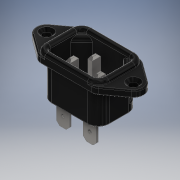
# Autodesk Inventor part: IEC C14
Saved by Autodesk Inventor 2017 SP1 (Build 210196100, 196)
## iProperties
Created: 2012-02-15
Part Number: IEC C14
Material: Tworzywo sztuczne, nieprzezroczyste czarne
Document SubType Name: Modeling
Designer: Ioannis
Density: 0.952 g/cm^3
Appearance: Gładkie - czarne
Author: Ioannis
Autodesk Inventor part; units mm, degrees
ref_plane "YZ Plane" through (0, 0, 0) normal (1, 0, 0) x (0, 1, 0)
ref_plane "XZ Plane" through (0, 0, 0) normal (0, 1, 0) x (-1, 0, 0)
ref_plane "XY Plane" through (0, 0, 0) normal (0, 0, 1) x (1, 0, 0)
sketch "Block1" plane through (0, 0, 0) normal (0, 0, 1) x (1, 0, 0)
  line L0 (24.7204, 7.7183) -> (30.7204, 7.7183)
  line L1 (30.7204, 7.7183) -> (30.7204, 9.1183)
  line L2 (29.2204, 14.6183) -> (26.2204, 14.6183)
  line L3 (24.7204, 9.1183) -> (24.7204, 7.7183)
  line L4 (26.2204, 14.6183) -> (24.7204, 9.1183)
  line L5 (30.7204, 9.1183) -> (29.2204, 14.6183)
  point P0 (27.9704, 11.8933)
  point P1 (30.7204, 14.6183)
  point P2 (24.7204, 14.6183)
  dimension "d122" = 6
  dimension "d123" = 6.9
  dimension "d124" = 1.5
  dimension "d125" = 5.5
  dimension "d126" = 5.5
  dimension "d127" = 1.5
  dimension "d128" = 6
  dimension "d130" = 105.255
  dimension "d131" = 105.255
  dimension "d132" = 1.4
  dimension "d133" = 1.4
  measures "d122" distance of point (24.72, 14.618) point (30.72, 14.618)
  measures "d123" distance of point (30.72, 14.618) L0.end
  measures "d124" distance of L2.end point (24.72, 14.618)
  measures "d125" distance of L3.start point (24.72, 14.618)
  measures "d126" distance of L1.end point (30.72, 14.618)
  measures "d127" distance of L2.start point (30.72, 14.618)
  measures "d128" distance of L0.start L0.end
  measures "d130" angle of L4 L2
  measures "d131" angle of L5 L2
  measures "d132" distance of L3.start L0.start
  measures "d133" distance of L0.end L1.end
sketch "Sketch1" plane through (0, 0, 0) normal (0, 0, 1) x (1, 0, 0)
  line L0 (-24.75, -11) -> (24.75, -11) construction
  line L1 (24.75, -11) -> (24.75, 11) construction
  line L2 (24.75, 11) -> (-24.75, 11) construction
  line L3 (-24.75, 11) -> (-24.75, -11) construction
  line L4 (-24.75, 0) -> (24.75, 0) construction
  circle A0 centre (-20, 0) radius 1.75 construction
  circle A1 centre (20, 0) radius 1.75 construction
  circle A2 centre (-20, 0) radius 4.75 construction
  circle A3 centre (20, 0) radius 4.75 construction
  line L5 (-14.0544, 10.2293) -> (-22.803, 3.8348)
  line L6 (22.803, 3.8348) -> (14.0544, 10.2293)
  line L7 (11.694, 11) -> (-11.694, 11)
  line L8 (-22.803, -3.8348) -> (-14.0544, -10.2293)
  line L9 (-11.694, -11) -> (11.694, -11)
  line L10 (14.0544, -10.2293) -> (22.803, -3.8348)
  arc A4 (-22.803, 3.8348) -> (-22.803, -3.8348) centre (-20, 0) ccw
  arc A5 (22.803, -3.8348) -> (22.803, 3.8348) centre (20, 0) ccw
  arc A6 (-11.694, 11) -> (-14.0544, 10.2293) centre (-11.694, 7) ccw
  arc A7 (14.0544, 10.2293) -> (11.694, 11) centre (11.694, 7) ccw
  arc A8 (11.694, -11) -> (14.0544, -10.2293) centre (11.694, -7) ccw
  arc A9 (-14.0544, -10.2293) -> (-11.694, -11) centre (-11.694, -7) ccw
  line L11 (9.875, -11) -> (-9.875, -11)
  line L12 (-14.875, -6) -> (-14.875, 6)
  line L13 (-9.875, 11) -> (9.875, 11)
  line L14 (14.875, 6) -> (14.875, -6)
  line L15 (9.875, -8.2) -> (-9.875, -8.2)
  line L16 (-12.075, -6) -> (-12.075, 6)
  line L17 (-9.875, 8.2) -> (9.875, 8.2)
  line L18 (12.075, 6) -> (12.075, -6)
  arc A10 (-9.875, 11) -> (-14.875, 6) centre (-9.875, 6) ccw
  arc A11 (14.875, 6) -> (9.875, 11) centre (9.875, 6) ccw
  arc A12 (-14.875, -6) -> (-9.875, -11) centre (-9.875, -6) ccw
  arc A13 (9.875, -11) -> (14.875, -6) centre (9.875, -6) ccw
  arc A14 (-9.875, 8.2) -> (-12.075, 6) centre (-9.875, 6) ccw
  arc A15 (12.075, 6) -> (9.875, 8.2) centre (9.875, 6) ccw
  arc A16 (9.875, -8.2) -> (12.075, -6) centre (9.875, -6) ccw
  arc A17 (-12.075, -6) -> (-9.875, -8.2) centre (-9.875, -6) ccw
  line L19 (-12.075, 6) -> (-9.875, 8.2)
  line L20 (12.075, 6) -> (9.875, 8.2)
  point P0 (0, 0)
  point P1 (0, 11)
  point P2 (13, 11)
  point P3 (-13, 11)
  point P4 (0, 11)
  point P5 (-13, -11)
  point P6 (13, -11)
  point P7 (0, -11)
  point P8 (0, -11)
  point P9 (0, 11)
  point P10 (14.875, 0)
  dimension "d0" = 49.5
  dimension "d1" = 22
  dimension "d2" = 3.5
  dimension "d3" = 3.5
  dimension "d4" = 4.75
  dimension "d5" = 4.75
  dimension "d6" = 40
  dimension "d7" = 26
  dimension "d8" = 26
  dimension "d9" = 4
  dimension "d10" = 4
  dimension "d11" = 4
  dimension "d12" = 4
  dimension "d13" = 2.8
  dimension "d14" = 5
  dimension "d15" = 5
  dimension "d16" = 2.2
  dimension "d17" = 2.2
  dimension "d18" = 2.2
  dimension "d19" = 2.2
  dimension "d20" = 29.75
  dimension "d21" = 24.15
  constraints: 42 end point, 34 point on circle, 28 tangent, 18 centre point, 10 perpendicular, 10 point on line, 8 midpoint, 6 coincident, 3 collinear, 2 equal radius, 2 horizontal, 2 horizontal alignment, 2 parallel, 2 vertical alignment, 3 other
  measures "d0" distance of L1.end L2.end
  measures "d1" distance of L2.end L0.start
  measures "d2" diameter of A1
  measures "d3" diameter of A0
  measures "d4" distance from line of L3 A0.centre
  measures "d5" distance from line of L1 A1.centre
  measures "d6" distance of A1.centre A0.centre
  measures "d7" distance of point (13, 11) point (-13, 11)
  measures "d8" distance of point (-13, -11) point (13, -11)
  measures "d9" radius of A6
  measures "d10" radius of A7
  measures "d11" radius of A8
  measures "d12" radius of A9
  measures "d13" distance between parallel lines of L14 L18
  measures "d14" radius of A10
  measures "d15" radius of A12
  measures "d16" radius of A14
  measures "d17" radius of A15
  measures "d18" radius of A16
  measures "d19" radius of A17
  measures "d20" distance between parallel lines of L14 L12
  measures "d21" distance between parallel lines of L18 L16
extrude "Extrusion1" add sketch "Sketch1" against normal blind 3.2 contours A6 L7 A10 L12 A12 L9 A9 L8 A4 L5 | L7 A11 L14 A13 L9 A12 L12 A10 | L7 A7 L6 A5 L10 A8 L9 A13 L14 A11 | L15 A17 L16 L19 L17 L20 L18 A16 | L20 A15 | A14 L19
extrude "Extrusion2" add sketch "Sketch1" along normal blind 1.8 contours L7 A11 L14 A13 L9 A12 L12 A10
sketch "Sketch2" plane through (0, 0, -3.2) normal (0, 0, -1) x (-1, 0, 0)
  line L0 (-12.075, -6) -> (-12.075, 6) projected
  arc A0 (-9.875, 8.2) -> (-12.075, 6) centre (-9.875, 6) ccw projected
  line L1 (-9.875, 8.2) -> (9.875, 8.2) projected
  arc A1 (12.075, 6) -> (9.875, 8.2) centre (9.875, 6) ccw projected
  line L2 (12.075, 6) -> (12.075, -6) projected
  arc A2 (9.875, -8.2) -> (12.075, -6) centre (9.875, -6) ccw projected
  line L3 (9.875, -8.2) -> (-9.875, -8.2) projected
  arc A3 (-12.075, -6) -> (-9.875, -8.2) centre (-9.875, -6) ccw projected
  line L4 (8.325, 9.45) -> (-8.325, 9.45)
  line L5 (-13.325, 4.45) -> (-13.325, -4.45)
  line L6 (-8.325, -9.45) -> (8.325, -9.45)
  line L7 (13.325, -4.45) -> (13.325, 4.45)
  arc A4 (-8.325, 9.45) -> (-13.325, 4.45) centre (-8.325, 4.45) ccw
  arc A5 (13.325, 4.45) -> (8.325, 9.45) centre (8.325, 4.45) ccw
  arc A6 (8.325, -9.45) -> (13.325, -4.45) centre (8.325, -4.45) ccw
  arc A7 (-13.325, -4.45) -> (-8.325, -9.45) centre (-8.325, -4.45) ccw
  point P0 (0, 0)
  dimension "d28" = 1.25
  dimension "d29" = 1.25
  dimension "d30" = 1.25
  dimension "d31" = 1.25
  dimension "d32" = 5
  dimension "d33" = 5
  dimension "d34" = 5
  dimension "d35" = 5
  constraints: 8 end point, 8 point on circle, 8 tangent, 4 centre point, 4 parallel
  measures "d28" distance between parallel lines of L0 L5
  measures "d29" distance between parallel lines of L4 L1
  measures "d30" distance between parallel lines of L3 L6
  measures "d31" distance between parallel lines of L2 L7
  measures "d32" radius of A4
  measures "d33" radius of A5
  measures "d34" radius of A6
  measures "d35" radius of A7
extrude "Extrusion4" add sketch "Sketch2" along normal blind 15 contours L0 A0 L1 A1 L2 A2 L3 A3 | A5 L7 A6 L6 A7 L5 A4 L4
extrude "Extrusion3" cut sketch "Sketch1" against normal blind 17.2 contours L15 A17 L16 L19 L17 L20 L18 A16 | L20 A15 | A14 L19
hole "Hole1" at (-20, 0, 0) at (20, 0, 0) direction (0, 0, -1) diameter 3.5 end through all countersink diameter 6 countersink angle 90
extrude "Extrusion5" add sketch "Sketch1" against normal up to surface (17.2 mm away) contours L20 A15 | A14 L19
move faces "Move Face1" translate (1.4142, -1.4142, 0) faces at (-11.3417, 6.7333, -5.7333) (10.6083, 7.4667, -5.7333)
move faces "Move Face2" translate (-1.4142, -1.4142, 0) faces at (10.6083, 7.4667, -5.7333)
ref_plane "Work Plane1" through (0, 0, -6.3) normal (0, 0, 1) x (1, 0, 0)
sketch "Sketch3" plane through (0, 0, -6.3) normal (0, 0, 1) x (1, 0, 0)
  line L0 (13.325, 5.125) -> (13.325, 9.45)
  line L1 (13.325, 9.45) -> (9, 9.45)
  line L2 (9, 9.45) -> (13.325, 5.125)
  line L3 (-9, 9.45) -> (-13.325, 9.45)
  line L4 (-13.325, 9.45) -> (-13.325, 5.125)
  line L5 (-13.325, 5.125) -> (-9, 9.45)
  line L6 (9, 9.45) -> (-9, 9.45) construction
  line L7 (8.325, 9.45) -> (-8.325, 9.45) construction
  line L8 (13.325, -4.45) -> (13.325, 4.45) construction
  line L9 (-13.325, 4.45) -> (-13.325, -4.45) construction
  point P0 (0, 0)
  point P1 (0, 9.45)
  dimension "d52" = 18
  dimension "d53" = 45
  dimension "d54" = 45
  constraints: 14 end point, 4 collinear, 3 perpendicular, 1 horizontal, 1 midpoint, 1 vertical, 1 vertical alignment
  measures "d52" distance of L3.start L1.end
  measures "d53" angle of L4 L5
  measures "d54" angle of L0 L2
extrude "Extrusion6" cut sketch "Sketch3" against normal blind 8
sketch "Sketch5" plane through (0, 0, -18.2) normal (0, 0, -1) x (-1, 0, 0)
  circle A0 centre (0, -2.45) radius 1.5
  arc A1 (13.325, 4.45) -> (8.325, 9.45) centre (8.325, 4.45) ccw projected
  line L0 (-8.325, 9.45) -> (8.325, 9.45) projected
  arc A2 (-8.325, 9.45) -> (-13.325, 4.45) centre (-8.325, 4.45) ccw projected
  line L1 (-13.325, -4.45) -> (-13.325, 4.45) projected
  arc A3 (-13.325, -4.45) -> (-8.325, -9.45) centre (-8.325, -4.45) ccw projected
  line L2 (8.325, -9.45) -> (-8.325, -9.45) projected
  arc A4 (8.325, -9.45) -> (13.325, -4.45) centre (8.325, -4.45) ccw projected
  line L3 (13.325, 4.45) -> (13.325, -4.45) projected
  line L4 (0, 9.45) -> (0, -9.45)
  line L5 (-7.75, 1.0821) -> (-4.75, 1.0821)
  line L6 (-4.75, 1.0821) -> (-3.75, -2.65)
  line L7 (-3.75, -2.65) -> (3.75, -2.65)
  line L8 (3.75, -2.65) -> (4.75, 1.0821)
  line L9 (4.75, 1.0821) -> (7.75, 1.0821)
  line L10 (8.325, -9.45) -> (-8.325, -9.45) projected
  line L11 (7.75, 2.5821) -> (3.599, 2.5821)
  line L12 (3.599, 2.5821) -> (2.599, -1.15)
  line L13 (2.599, -1.15) -> (-2.599, -1.15)
  line L14 (-2.599, -1.15) -> (-3.599, 2.5821)
  line L15 (-3.599, 2.5821) -> (-7.75, 2.5821)
  line L16 (-7.75, 1.0821) -> (-7.75, 2.5821)
  line L17 (7.75, 2.5821) -> (7.75, 1.0821)
  point P0 (0, 0)
  point P1 (0, -2.65)
  dimension "d104" = 3
  dimension "d105" = 7
  dimension "d106" = 105
  dimension "d107" = 105
  dimension "d108" = 7.5
  dimension "d109" = 15.5
  dimension "d110" = 6.8
  dimension "d111" = 3
  dimension "d112" = 3.7321
  dimension "d113" = 1.5
  constraints: 26 end point, 5 collinear, 4 midpoint, 4 parallel, 2 perpendicular, 2 vertical alignment, 1 centre point, 4 other
  measures "d104" diameter of A0
  measures "d105" distance from line of L2 A0.centre
  measures "d106" angle of L7 L6
  measures "d107" angle of L8 L7
  measures "d108" distance of L6.end L7.end
  measures "d109" distance of L5.start L9.end
  measures "d110" distance between parallel lines of L2 L7
  measures "d111" distance of L5.start L5.end
  measures "d112" distance between parallel lines of L7 L5
  measures "d113" distance between parallel lines of L11 L9
extrude "Extrusion9" add sketch "Sketch5" along normal blind 3.4 contours A0 L7 L4 L13 | A0 L13 L12 L11 L17 L9 L8 L7 | L13 L4 A0 | A0 L4 L7 | L4 L13 A0 | L4 L7 A0 L13 | A0 L7 L4 | A0 L7 L6 L5 L16 L15 L14 L13
fillet "Fillet2" radius 0.5 38 edges at (0, 9.45, -18.2) (-11.8605, 7.9855, -18.2) (-13.325, 0, -18.2) (-11.8605, -7.9855, -18.2) (0, -9.45, -18.2) (11.8605, -7.9855, -18.2) (13.325, 0, -18.2) (11.8605, 7.9855, -18.2) (-10.7845, 11, 0) (-18.4287, 7.0321, 0) (-24.75, 0, 0) (-18.4287, -7.0321, 0) (-12.9355, -10.8025, 0) (-10.7845, -11, 0) (-12.9355, 10.8025, 0) (24.75, 0, 0) (18.4287, -7.0321, 0) (12.9355, -10.8025, 0) (10.7845, -11, 0) (12.9355, 10.8025, 0) (10.7845, 11, 0) (18.4287, 7.0321, 0) (-11.8605, 7.9855, -14.3) (-11.8605, 7.9855, -6.3) (11.8605, 7.9855, -14.3) (11.8605, 7.9855, -6.3) (12.9355, -10.8025, -3.2) (18.4287, -7.0321, -3.2) (24.75, 0, -3.2) (18.4287, 7.0321, -3.2) (12.9355, 10.8025, -3.2) (0, 11, -3.2) (-12.9355, 10.8025, -3.2) (-18.4287, 7.0321, -3.2) (-24.75, 0, -3.2) (-18.4287, -7.0321, -3.2) (-12.9355, -10.8025, -3.2) (0, -11, -3.2)
full round fillet "Fillet1" first side at (2.0417, 11, -1.9667) (14.875, 0.1239, 1.2) (11.5825, 10.6994, 1.1915) (-10.5207, 10.9581, 1.1168) (-14.875, 2, 0.6) (-10.5207, -10.9581, 1.1168) (2.0417, -11, -1.9667) (10.5207, -10.9581, 1.1168) centre faces at (-1.795, 10.0667, 1.8) second side at (1.795, 8.2, -12.9118)
fillet "Fillet3" radius 2 2 edges at (-9.5608, 5.6858, 0) (9.5608, 5.6858, 0)
sketch "Sketch4" plane through (0, 0, -17.2) normal (0, 0, 1) x (1, 0, 0)
  line L0 (8.325, 8.95) -> (-8.325, 8.95) projected
  arc A0 (12.825, 4.45) -> (8.325, 8.95) centre (8.325, 4.45) ccw projected
  line L1 (12.825, -4.45) -> (12.825, 4.45) projected
  arc A1 (8.325, -8.95) -> (12.825, -4.45) centre (8.325, -4.45) ccw projected
  line L2 (-8.325, -8.95) -> (8.325, -8.95) projected
  arc A2 (-12.825, -4.45) -> (-8.325, -8.95) centre (-8.325, -4.45) ccw projected
  line L3 (-12.825, 4.45) -> (-12.825, -4.45) projected
  arc A3 (-8.325, 8.95) -> (-12.825, 4.45) centre (-8.325, 4.45) ccw projected
  line L4 (-8.8, 1.05) -> (-3.6, 1.05)
  line L5 (-3.6, 1.05) -> (-3.6, -8.95)
  line L6 (-3.6, -8.95) -> (-8.8, -8.95)
  line L7 (-8.8, -8.95) -> (-8.8, 1.05)
  line L8 (3.6, 1.05) -> (8.8, 1.05)
  line L9 (8.8, 1.05) -> (8.8, -8.95)
  line L10 (8.8, -8.95) -> (3.6, -8.95)
  line L11 (3.6, -8.95) -> (3.6, 1.05)
  line L12 (2.6, -1.05) -> (-2.6, -1.05)
  line L13 (-2.6, -1.05) -> (-2.6, 8.95)
  line L14 (-2.6, 8.95) -> (2.6, 8.95)
  line L15 (2.6, 8.95) -> (2.6, -1.05)
  line L16 (-6.2, 1.05) -> (-6.2, -8.95) construction
  line L17 (0, 8.95) -> (0, -1.05) construction
  line L18 (6.2, 1.05) -> (6.2, -8.95) construction
  line L19 (-5.2, -3.95) -> (-7.2, -3.95)
  line L20 (-7.2, -3.95) -> (-7.2, 0.05)
  line L21 (-7.2, 0.05) -> (-5.2, 0.05)
  line L22 (-5.2, 0.05) -> (-5.2, -3.95)
  line L23 (7.2, 0.05) -> (5.2, 0.05)
  line L24 (5.2, 0.05) -> (5.2, -3.95)
  line L25 (5.2, -3.95) -> (7.2, -3.95)
  line L26 (7.2, -3.95) -> (7.2, 0.05)
  line L27 (1, -0.05) -> (-1, -0.05)
  line L28 (-1, -0.05) -> (-1, 3.95)
  line L29 (-1, 3.95) -> (1, 3.95)
  line L30 (1, 3.95) -> (1, -0.05)
  point P0 (0, 0)
  point P1 (-6.2, -1.95)
  point P2 (-6.2, 0.05)
  point P3 (-5.2, -1.95)
  point P4 (6.2, -1.95)
  point P5 (6.2, -3.95)
  point P6 (7.2, -1.95)
  point P7 (0, 1.95)
  point P8 (0, 3.95)
  point P9 (1, 1.95)
  dimension "d57" = 1
  dimension "d58" = 1
  dimension "d59" = 5.2
  dimension "d60" = 5.2
  dimension "d61" = 5.2
  dimension "d62" = 4.025
  dimension "d63" = 4.025
  dimension "d64" = 10
  dimension "d65" = 10
  dimension "d66" = 4
  dimension "d67" = 2
  dimension "d68" = 1
  dimension "d69" = 2
  dimension "d70" = 4
  dimension "d71" = 1
  dimension "d72" = 2
  dimension "d73" = 4
  dimension "d74" = 1
  constraints: 54 end point, 19 perpendicular, 13 midpoint, 6 horizontal, 5 point on line, 3 horizontal alignment, 3 vertical alignment, 1 collinear, 1 parallel
  measures "d57" distance between parallel lines of L11 L15
  measures "d58" distance between parallel lines of L5 L13
  measures "d59" distance of L12.start L12.end
  measures "d60" distance of L8.start L8.end
  measures "d61" distance of L4.start L4.end
  measures "d62" distance between parallel lines of L1 L9
  measures "d63" distance between parallel lines of L3 L7
  measures "d64" distance of L14.end L12.start
  measures "d65" distance of L10.end L8.start
  measures "d66" distance of L19.end L20.end
  measures "d67" distance of L19.start L19.end
  measures "d68" distance between parallel lines of L4 L21
  measures "d69" distance of L23.start L23.end
  measures "d70" distance of L25.end L23.start
  measures "d71" distance between parallel lines of L8 L23
  measures "d72" distance of L28.end L29.end
  measures "d73" distance of L27.end L28.end
  measures "d74" distance between parallel lines of L12 L27
extrude "Extrusion7" add sketch "Sketch4" along normal blind 2.5 contours L15 L12 L13 L0 | L9 L10 A1 | A1 L2 L11 L8 L9 | L7 L4 L5 L2 A2 | A2 L6 L7
extrude "Extrusion8" add sketch "Sketch4" along normal blind 15 contours L19 L20 L21 L22 | L26 L25 L24 L23 | L27 L28 L29 L30
move faces "Move Face3" translate (0, 0, 2) faces at (-0.3333, 2.6167, -2.2)
chamfer "Chamfer1" distance 1 angle 30 1 edges at (-1, 1.95, -0.2) measured on face at (-1, 1.95, -0.7)
chamfer "Chamfer4" distance 1 angle 30 1 edges at (1, 1.95, -0.2) measured on face at (1, 1.95, -0.7)
chamfer "Chamfer5" distance 1 angle 30 1 edges at (5.2, -1.95, -2.2) measured on face at (5.2, -1.95, -2.7)
chamfer "Chamfer6" distance 1 angle 30 1 edges at (7.2, -1.95, -2.2) measured on face at (7.2, -1.95, -2.7)
chamfer "Chamfer7" distance 1 angle 30 1 edges at (-5.2, -1.95, -2.2) measured on face at (-5.2, -1.95, -2.7)
chamfer "Chamfer8" distance 1 angle 30 1 edges at (-7.2, -1.95, -2.2) measured on face at (-7.2, -1.95, -2.7)
chamfer "Chamfer2" distance 1 angle 45 6 edges at (0, 3.95, -0.2) (0, -0.05, -0.2) (-6.2, 0.05, -2.2) (-6.2, -3.95, -2.2) (6.2, 0.05, -2.2) (6.2, -3.95, -2.2)
sketch "Sketch6" plane through (0, 0, -18.2) normal (0, 0, -1) x (-1, 0, 0)
  line L0 (1, -0.05) -> (1, 3.95) projected
  line L1 (1, 3.95) -> (-1, 3.95) projected
  line L2 (-1, 3.95) -> (-1, -0.05) projected
  line L3 (-1, -0.05) -> (1, -0.05) projected
  line L4 (7.2, -3.95) -> (7.2, 0.05) projected
  line L5 (7.2, 0.05) -> (5.2, 0.05) projected
  line L6 (5.2, 0.05) -> (5.2, -3.95) projected
  line L7 (5.2, -3.95) -> (7.2, -3.95) projected
  line L8 (-7.2, 0.05) -> (-7.2, -3.95) projected
  line L9 (-7.2, -3.95) -> (-5.2, -3.95) projected
  line L10 (-5.2, -3.95) -> (-5.2, 0.05) projected
  line L11 (-5.2, 0.05) -> (-7.2, 0.05) projected
  line L12 (9.2, -5.4179) -> (3.2, -5.4179)
  line L13 (3.2, -5.4179) -> (3.2, -6.3179)
  line L14 (3.2, -6.3179) -> (9.2, -6.3179)
  line L15 (9.2, -6.3179) -> (9.2, -5.4179)
  line L16 (-9.2, -5.4179) -> (-3.2, -5.4179)
  line L17 (-3.2, -5.4179) -> (-3.2, -6.3179)
  line L18 (-3.2, -6.3179) -> (-9.2, -6.3179)
  line L19 (-9.2, -6.3179) -> (-9.2, -5.4179)
  line L20 (3, 6.25) -> (-3, 6.25)
  line L21 (-3, 6.25) -> (-3, 5.35)
  line L22 (-3, 5.35) -> (3, 5.35)
  line L23 (3, 5.35) -> (3, 6.25)
  line L24 (7.75, 1.0821) -> (4.75, 1.0821) projected
  line L25 (-2.599, -1.15) -> (-0.7483, -1.15) projected
  line L26 (-4.75, 1.0821) -> (-7.75, 1.0821) projected
  line L27 (3.2, -6.3179) -> (9.2, -6.3179)
  line L28 (9.2, -6.3179) -> (9.2, -4.9179)
  line L29 (7.7, 0.5821) -> (4.7, 0.5821)
  line L30 (3.2, -4.9179) -> (3.2, -6.3179)
  line L31 (4.7, 0.5821) -> (3.2, -4.9179)
  line L32 (9.2, -4.9179) -> (7.7, 0.5821)
  line L33 (-9.2, -6.3179) -> (-3.2, -6.3179)
  line L34 (-3.2, -6.3179) -> (-3.2, -4.9179)
  line L35 (-4.7, 0.5821) -> (-7.7, 0.5821)
  line L36 (-9.2, -4.9179) -> (-9.2, -6.3179)
  line L37 (-7.7, 0.5821) -> (-9.2, -4.9179)
  line L38 (-3.2, -4.9179) -> (-4.7, 0.5821)
  line L39 (3, 6.25) -> (-3, 6.25)
  line L40 (-3, 6.25) -> (-3, 4.85)
  line L41 (-1.5, -0.65) -> (1.5, -0.65)
  line L42 (3, 4.85) -> (3, 6.25)
  line L43 (1.5, -0.65) -> (3, 4.85)
  line L44 (-3, 4.85) -> (-1.5, -0.65)
  point P0 (0, 0)
  point P1 (6.2, -3.95)
  point P2 (-6.2, -3.95)
  point P3 (0, 3.95)
  point P4 (6.2, -6.3179)
  point P5 (6.2, 0.5821)
  point P6 (6.2, -6.3179)
  point P7 (6.2, -6.3179)
  point P8 (6.2, -6.3179)
  point P9 (0, 6.25)
  point P10 (0, 6.25)
  point P11 (-6.2, -6.3179)
  point P12 (-6.2, -6.3179)
  point P13 (-6.2, -6.3179)
  dimension "d116" = 6
  dimension "d117" = 6
  dimension "d118" = 6
  dimension "d119" = 0.9
  dimension "d120" = 0.9
  dimension "d121" = 0.9
  dimension "d134" = 0.5
  dimension "d135" = 0.5
  dimension "d136" = 0.5
  constraints: 24 end point, 9 perpendicular, 6 midpoint, 3 coincident, 3 horizontal, 3 vertical alignment, 1 collinear, 7 other
  measures "d116" distance of L13.end L14.end
  measures "d117" distance of L17.end L18.end
  measures "d118" distance of L21.end L22.end
  measures "d119" distance of L14.end L12.start
  measures "d120" distance of L16.end L17.end
  measures "d121" distance of L22.end L20.start
extrude "Extrusion10" add sketch "Sketch6" along normal blind 0.9 contours L3 L2 L1 L0 | L7 L6 L5 L4 | L11 L10 L9 L8 | L12 L30 L31 L29 L32 L28 | L36 L37 L35 L38 L34 L16 | L42 L43 L41 L44 L40 L22
extrude "Extrusion11" add sketch "Sketch6" along normal blind 10 contours L15 L14 L13 L12 | L16 L17 L18 L19 | L23 L22 L21 L20
sketch "Sketch7" plane through (-8.325, -9.45, -3.2) normal (0, -1, 0) x (1, 0, 0)
  circle A0 centre (8.325, -20.3) radius 0.75
  circle A1 centre (2.125, -20.3) radius 0.75
  circle A2 centre (14.525, -20.3) radius 0.75
  line L0 (21.5145, -20.3) -> (-4.8645, -20.3) construction
  line L1 (11.525, -25) -> (17.525, -25) projected
  line L2 (-0.875, -25) -> (5.125, -25) projected
  point P0 (8.325, 3.2)
  point P1 (14.525, -25)
  point P2 (2.125, -25)
  dimension "d141" = 1.5
  dimension "d142" = 1.5
  dimension "d143" = 1.5
  dimension "d144" = 4.7
  dimension "d145" = 6.2
  dimension "d147" = 6.2
  constraints: 3 centre point, 3 midpoint, 2 end point, 2 point on line, 2 vertical alignment, 1 coincident, 1 horizontal
  measures "d141" diameter of A2
  measures "d142" diameter of A0
  measures "d143" diameter of A1
  measures "d144" distance between parallel lines of L0 L1
  measures "d145" distance of A0.centre A2.centre
  measures "d147" distance of A0.centre A1.centre
extrude "Extrusion12" cut sketch "Sketch7" against normal through all
chamfer "Chamfer9" distance 1.5 angle 45 6 edges at (-3, 5.8, -28.2) (3, 5.8, -28.2) (3.2, -5.8679, -28.2) (9.2, -5.8679, -28.2) (-3.2, -5.8679, -28.2) (-9.2, -5.8679, -28.2)
equation "\"d2\" = d3"
equation "\"d5\" = d4"
equation "\"d9\" = d10"
equation "\"d11\" = d12"
equation "\"d12\" = d10"
equation "\"d29\" = d28"
equation "\"d30\" = d28"
equation "\"d31\" = d28"
equation "\"d54\" = d53"
equation "\"d107\" = d106"
equation "\"d58\" = d57"
equation "\"d60\" = d61"
equation "\"d61\" = d59"
equation "\"d62\" = d63"
equation "\"d65\" = d64"
equation "\"d69\" = d67"
equation "\"d70\" = d66"
equation "\"d71\" = d68"
equation "\"d72\" = d67"
equation "\"d73\" = d66"
equation "\"d74\" = d68"
equation "\"d117\" = d116"
equation "\"d118\" = d117"
equation "\"d120\" = d119"
equation "\"d121\" = d119"
equation "\"d135\" = d134"
equation "\"d142\" = d141"
equation "\"d143\" = d142"
equation "\"d145\" = d147"
equation "\"d124\" = d127"
equation "\"d126\" = d125"
body "Solid1"
